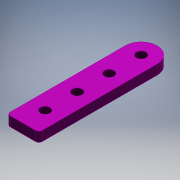
# Autodesk Inventor part: Slider_1_spacer
Saved by Autodesk Inventor 2016 (Build 200138000, 138)
## iProperties
Created: 2015-12-09
Part Number: Slider_1_spacer
Material: Generic
Document SubType Name: Modeling
Designer: lk8187
Density: 1 g/cm^3
Appearance: Smooth - Purple
Author: lk8187
Autodesk Inventor part; units mm, degrees
ref_plane "YZ Plane" through (0, 0, 0) normal (1, 0, 0) x (0, 1, 0)
ref_plane "XZ Plane" through (0, 0, 0) normal (0, 1, 0) x (-1, 0, 0)
ref_plane "XY Plane" through (0, 0, 0) normal (0, 0, 1) x (1, 0, 0)
sketch "Sketch1" plane through (0, 0, 0) normal (0, 0, 1) x (1, 0, 0)
  line L0 (0, 0) -> (0, 20) construction
  line L1 (5, 0) -> (5, 20)
  line L2 (-5, 20) -> (-5, 19.2786)
  arc A0 (5, 20) -> (-5, 20) centre (0, 20) ccw
  circle A1 centre (0, 20) radius 1.5
  circle A2 centre (0, 10) radius 1.5
  circle A3 centre (0, 0) radius 1.5
  line L3 (-5, 19.2786) -> (-5, -16)
  line L4 (-4, -17) -> (4, -17)
  line L5 (5, -16) -> (5, 0)
  arc A4 (-5, -16) -> (-4, -17) centre (-4, -16) ccw
  arc A5 (4, -17) -> (5, -16) centre (4, -16) ccw
  circle A6 centre (0, -10) radius 1.5
  dimension "d0" = 10
  dimension "d1" = 20
  dimension "d2" = 3
  dimension "d5" = 1
  dimension "d6" = 17
  dimension "d7" = 3
  dimension "d8" = 10
  constraints: 14 end point, 7 centre point, 6 point on circle, 6 tangent, 3 coincident, 3 equal radius, 2 perpendicular, 2 vertical, 1 collinear, 1 horizontal alignment, 1 midpoint, 1 parallel, 1 vertical alignment
  measures "d0" distance between parallel lines of L1 L2
  measures "d1" distance of L0.start L0.end
  measures "d2" diameter of A2
  measures "d5" radius of A4
  measures "d6" distance from line of L4 L0.start
  measures "d7" diameter of A6
  measures "d8" distance of A6.centre L0.start
extrude "Extrusion1" add sketch "Sketch1" along normal blind 3
body "Solid1"
